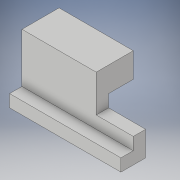
# Autodesk Inventor part: Model Creation 4
Saved by Autodesk Inventor 2019 (Build 230136000, 136)
## iProperties
Created: 2019-09-09
Part Number: Model Creation 4
Material: Generic
Document SubType Name: Modeling
Designer: IED8
Density: 1 g/cm^3
Appearance: Default
Author: IED8
Autodesk Inventor part; units mm, degrees
ref_plane "YZ Plane" through (0, 0, 0) normal (1, 0, 0) x (0, 1, 0)
ref_plane "XZ Plane" through (0, 0, 0) normal (0, 1, 0) x (-1, 0, 0)
ref_plane "XY Plane" through (0, 0, 0) normal (0, 0, 1) x (1, 0, 0)
sketch "Sketch1" plane through (0, 0, 0) normal (1, 0, 0) x (0, 1, 0)
  line L0 (0, 0) -> (0, -25.4)
  line L1 (0, -25.4) -> (38.1, -25.4)
  line L2 (38.1, -25.4) -> (38.1, -50.8)
  line L3 (38.1, -50.8) -> (63.5, -50.8)
  line L4 (63.5, -50.8) -> (63.5, -12.7)
  line L5 (63.5, -12.7) -> (12.7, -12.7)
  line L6 (12.7, -12.7) -> (12.7, 0)
  line L7 (12.7, 0) -> (0, 0)
  dimension "d0" = 25.4
  dimension "d1" = 38.1
  dimension "d2" = 25.4
  dimension "d3" = 25.4
  dimension "d4" = 38.1
  dimension "d5" = 50.8
  constraints: 16 end point, 5 perpendicular, 2 vertical, 1 horizontal
  measures "d0" distance of L0.start L0.end
  measures "d1" distance of L0.end L1.end
  measures "d2" distance of L1.end L2.end
  measures "d3" distance of L2.end L3.end
  measures "d4" distance of L3.end L4.end
  measures "d5" distance of L4.end L5.end
extrude "Extrusion1" add sketch "Sketch1" along normal blind 114.3
sketch "Sketch2" plane through (114.3, 0, 0) normal (1, 0, 0) x (0, 0, -1)
  line L0 (50.8, 38.1) -> (50.8, 63.5) projected
  line L1 (50.8, 38.1) -> (50.8, 63.5)
  line L2 (50.8, 63.5) -> (12.7, 63.5) projected
  line L3 (50.8, 63.5) -> (12.7, 63.5)
  line L4 (12.7, 63.5) -> (12.7, 25.4)
  line L5 (12.7, 63.5) -> (12.7, 12.7) projected
  line L6 (12.7, 25.4) -> (25.4, 25.4)
  line L7 (25.4, 0) -> (25.4, 38.1) projected
  line L8 (25.4, 25.4) -> (25.4, 38.1)
  line L9 (25.4, 38.1) -> (50.8, 38.1)
  point P0 (0, 0)
  dimension "d8" = 38.1
  constraints: 12 end point, 3 collinear, 2 perpendicular, 2 point on line
  measures "d8" distance of L2.end L4.end
extrude "Extrusion2" cut sketch "Sketch2" against normal blind 38.1
body "Solid1"
